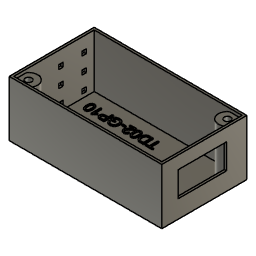
TD02-GP10 (Autodesk Fusion 360 archive; units mm, degrees)
design "boite"
Autodesk Fusion 360 part; units mm, degrees
note: some values were not read from the file. Chosen so that the rebuilt part matches the saved one: that a step has no effect; which face or edge a step refers to; which pieces of a blend or face edit are solid. Set by a fixed rule: which sketch regions a step uses.
sketch "Sketch1" plane through (0, 0, 0) normal (0, 0, 1) x (1, 0, 0)
  line L0 (-39.5, 22) -> (39.5, 22)
  line L1 (39.5, 22) -> (39.5, -22)
  line L2 (39.5, -22) -> (-39.5, -22)
  line L3 (-39.5, -22) -> (-39.5, 22)
  line L4 (-39.5, 22) -> (39.5, -22) construction
  line L5 (39.5, 22) -> (-39.5, -22) construction
  line L6 (38.3, -20.8) -> (-38.3, -20.8)
  line L7 (-38.3, -20.8) -> (-38.3, 20.8)
  line L8 (-38.3, 20.8) -> (38.3, 20.8)
  line L9 (38.3, 20.8) -> (38.3, -20.8)
  line L10 (-37.5, 20) -> (37.5, 20) construction
  line L11 (37.5, 20) -> (37.5, -20) construction
  line L12 (37.5, -20) -> (-37.5, -20) construction
  line L13 (-37.5, -20) -> (-37.5, 20) construction
  line L14 (-37.5, 20) -> (37.5, -20) construction
  line L15 (37.5, 20) -> (-37.5, -20) construction
  line L16 (-37.5, 20) -> (-34.5, 20) construction
  line L17 (-34.5, 20) -> (-34.5, 17) construction
  line L18 (-34.5, 17) -> (-37.5, 17) construction
  line L19 (-37.5, 17) -> (-37.5, 20) construction
  circle A0 centre (-34.5, 17) radius 2.9
  line L20 (37.5, -20) -> (34.5, -20) construction
  line L21 (34.5, -20) -> (34.5, -17) construction
  line L22 (34.5, -17) -> (37.5, -17) construction
  line L23 (37.5, -17) -> (37.5, -20) construction
  circle A1 centre (34.5, -17) radius 2.9
  circle A2 centre (-34.5, 17) radius 3.7
  circle A3 centre (34.5, -17) radius 3.7
  circle A4 centre (-34.5, 17) radius 1.7
  circle A5 centre (34.5, -17) radius 1.7
  line L24 (20, 0) -> (2.5, 0)
  circle A6 centre (-34.5, -17) radius 3.7
  circle A7 centre (-34.5, -17) radius 2.9
  circle A8 centre (-34.5, -17) radius 1.7
  circle A9 centre (34.5, 17) radius 3.7
  circle A10 centre (34.5, 17) radius 2.9
  circle A11 centre (34.5, 17) radius 1.7
  circle A12 centre (34.5, 17) radius 4.7
  circle A13 centre (-34.5, -17) radius 4.7
  dimension "d1" = 79
  dimension "d2" = 44
  dimension "d3" = 1.2
  dimension "d4" = 75
  dimension "d5" = 40
  dimension "d6" = 3
  dimension "d7" = 3
  dimension "d8" = 5.8
  dimension "d10" = 3
  dimension "d11" = 3
  dimension "d12" = 5.8
  dimension "d32" = 0.8
  dimension "d33" = 0.8
  dimension "d44" = 3.4
  dimension "d45" = 3.4
  dimension "d90" = 1
  dimension "d91" = 1
  constraint horizontal L0
  constraint perpendicular L0 L1
  constraint parallel L0 L2
  constraint parallel L1 L3
  constraint coincident L4 origin
  constraint coincident L5 origin
  constraint horizontal L10
  constraint perpendicular L10 L11
  constraint parallel L10 L12
  constraint parallel L11 L13
  constraint coincident L14 origin
  constraint coincident L15 origin
  constraint horizontal L16
  constraint vertical L17
  constraint horizontal L18
  constraint vertical L19
  constraint coincident L17.end L18.start
  constraint horizontal L20
  constraint vertical L21
  constraint horizontal L22
  constraint vertical L23
  constraint coincident L21.end L22.start
  constraint concentric A0 A4
  constraint concentric A1 A5
  constraint symmetric A0 L24 A7
  constraint symmetric A1 L24 A10
  constraint symmetric A2 L24 A6
  constraint symmetric A3 L24 A9
  constraint symmetric A4 L24 A8
  constraint symmetric A5 L24 A11
  measures "d1" distance of L0.start L0.end
  measures "d2" distance of L0.start L2.end
  measures "d4" distance of L11.end L12.end
  measures "d5" distance of L10.start L12.end
  measures "d6" distance of L10.start L16.end
  measures "d7" distance of L16.end L17.end
  measures "d8" diameter of A0
  measures "d10" distance of L11.end L22.end
  measures "d11" distance of L21.end L22.end
  measures "d12" diameter of A1
  measures "d44" diameter of A4
  measures "d45" diameter of A5
extrude "Extrude7" [no effect]
extrude "Extrude9" add sketch "Sketch1" against normal blind 1.2 contours L0 L1 L2 L3 | L6 L7 L8 L9 A12 A13 | L6 A13 | L6 L7 A13 | L8 L9 A12 | L9 A12 | L6 L7 A13 | L8 L9 A12 | L8 A12 | L7 A13 | A2 | A3 | A6 | A7 | A8 | A9 | A10 | A11
extrude "Extrude10" add sketch "Sketch1" along normal blind 27.6 contours L0 L1 L2 L3 | L6 A13 | L9 A12 | L8 A12 | L7 A13 | A0 | A1 | A2 | A3 | A4 | A5
extrude "Extrude11" cut sketch "Sketch1" along normal blind 21.6 contours A1 | A5
extrude "Extrude12" cut sketch "Sketch1" along normal blind 22.2 contours A0 | A4
extrude "Extrude13" cut 1 faces at (33.7592, -18.0865, 21.6) along direction (0, 0, 1) blind 0.6
extrude "Extrude14" cut sketch "Sketch1" along normal blind 40 contours A5
extrude "Extrude15" cut sketch "Sketch1" along normal blind 34 contours A4
extrude "Extrude16" cut sketch "Sketch1" along normal mid plane 100 contours A11
extrude "Extrude17" add sketch "Sketch1" along normal blind 27.6 contours A9 | A10
extrude "Extrude18" cut sketch "Sketch1" against normal blind 6 contours A10
extrude "Extrude19" cut sketch "Sketch1" along normal blind 22.2 contours A10
extrude "Extrude20" cut sketch "Sketch1" along normal mid plane 92 contours A8
extrude "Extrude21" add sketch "Sketch1" along normal blind 26.6 contours A6 | A7
extrude "Extrude22" cut sketch "Sketch1" along normal blind 22.2 contours A7
extrude "Extrude23" cut sketch "Sketch1" against normal blind 3 contours A7
delete_face "DeleteFace1" 1 faces at (-32.0171, 16.7715, 22.2)
delete_face "DeleteFace2" 6 faces at (-30.8184, 17.3684, 10.2757) (-30.8184, 17.3684, 19.4757) (-31.0912, 16.6721, 27.6) (-31.6144, 17.2887, 25.8) (-31.6144, 17.2887, 17.6757) (-31.6144, 17.2887, 10.2757)
delete_face "DeleteFace3" 1 faces at (-31.6036, 16.8554, -0.8)
delete_face "DeleteFace4" 1 faces at (38.1954, -17.1844, 18.4)
delete_face "DeleteFace5" 1 faces at (37.3964, -17.1446, -0.8)
sketch "Sketch3" plane through (39.5, 0, 0) normal (1, 0, 0) x (0, 1, 0)
  line L0 (-22, 27.6) -> (-22, -1.2) construction
  line L1 (-22, -1.2) -> (22, -1.2) construction
  line L2 (22, -1.2) -> (22, 27.6) construction
  line L3 (22, 27.6) -> (-22, 27.6) construction
  line L4 (-22, 27.6) -> (-9, 27.6) construction
  line L5 (-9, 27.6) -> (-9, 16.6) construction
  line L6 (-9, 16.6) -> (-22, 16.6) construction
  line L7 (-22, 16.6) -> (-22, 27.6) construction
  circle A0 centre (-12, 19.8) radius 4.3863
  line L8 (-7.9908, 18.0207) -> (-11.9971, 8.9935)
  line L9 (-11.9971, 8.9935) -> (-16.0083, 18.0185)
  dimension "d66" = 13
  dimension "d67" = 11
  dimension "d68" = 9.8762
  constraint horizontal L4
  constraint vertical L5
  constraint horizontal L6
  constraint vertical L7
  constraint coincident L0.start L3.end
  constraint coincident L5.end A0
  constraint coincident A0 L8.start
  constraint coincident A0 L9.end
  constraint tangent A0 L9
  constraint tangent A0 L8
  measures "d66" distance of L0.start L4.end
  measures "d67" distance of L4.end L5.end
  measures "d68" distance of L8.start L8.end
move_body "Move1" bodies 1 to x (1, 0, 0) y (0, 1, 0) z (0, 0, 1) at (0, -5.5, 0)
move_body "Move2" bodies 1 to x (1, 0, 0) y (0, 1, 0) z (0, 0, 1) at (0, 3, 0)
extrude "Extrude24" cut sketch "Sketch3" against normal blind 14
extrude "Extrude25" cut 1 faces at (-31.4868, -19.7683, 26.6) along direction (0, 0, -1) blind 0.6
extrude "Extrude26" cut 1 faces at (37.5132, 14.2317, 27.6) along direction (0, 0, -1) blind 1.6
delete_face "DeleteFace6" 2 faces at (39.1, -16.1636, 18.4201) (39.1, -9.3262, 15.0116)
sketch "Sketch4" plane through (39.5, 0, 0) normal (1, 0, 0) x (0, 1, 0)
  line L0 (19.5, 27.6) -> (-24.5, 27.6)
  line L1 (-24.5, 27.6) -> (-24.5, -1.2)
  line L2 (-24.5, -1.2) -> (19.5, -1.2)
  line L3 (19.5, -1.2) -> (19.5, 27.6)
  line L4 (9, 8) -> (-16, 8)
  line L5 (-16, 8) -> (-16, 21)
  line L6 (-16, 21) -> (9, 21)
  line L7 (9, 21) -> (9, 8)
  constraint horizontal L4
  constraint vertical L5
  constraint horizontal L6
  constraint vertical L7
extrude "Extrude27" cut sketch "Sketch4" against normal blind 16 contours L4 L5 L6 L7
sketch "Sketch5" plane through (0, 0, -1.2) normal (0, 0, -1) x (1, 0, 0)
  circle A0 centre (-34.5, 19.5) radius 2.9
  circle A1 centre (34.5, -14.5) radius 2.9
  line L0 (39.5, 24.5) -> (-39.5, 24.5)
  line L1 (-39.5, 24.5) -> (-39.5, -19.5)
  line L2 (-39.5, -19.5) -> (39.5, -19.5)
  line L3 (39.5, -19.5) -> (39.5, 24.5)
  circle A2 centre (23, 13) radius 7.6158
extrude "Extrude28" cut sketch "Sketch5" against normal blind 5 contours A2
sketch "Sketch6" plane through (0, 0, 0) normal (0, 0, 1) x (-1, 0, 0)
  circle A0 centre (-23, 13) radius 7.6158
  circle A1 centre (34.5, 19.5) radius 3.7
  circle A2 centre (-34.5, -14.5) radius 3.7
  line L0 (38.3, -18.3) -> (38.3, 23.3)
  line L1 (38.3, 23.3) -> (-38.3, 23.3)
  line L2 (-38.3, 23.3) -> (-38.3, -18.3)
  line L3 (-38.3, -18.3) -> (38.3, -18.3)
  line L4 (-3.0028, -22.2598) -> (29.9972, -22.2598) construction
  line L5 (29.9972, -22.2598) -> (29.9972, -7.2598) construction
  line L6 (29.9972, -7.2598) -> (-3.0028, -7.2598) construction
  line L7 (-3.0028, -7.2598) -> (-3.0028, -22.2598) construction
  dimension "d79" = 5
  text T0 "TD02-GP10\n" font "Arial" height 5 align left top in box 33 x 15 at (-3.0028, -22.2598) x (1, 0) y (0, 1) spacing 1
extrude "Extrude29" add sketch "Sketch6" along normal blind 0.4 text T0
sketch "Sketch7" plane through (-39.5, 0, 0) normal (-1, 0, 0) x (0, -1, 0)
  line L0 (-19.5, 27.6) -> (-19.5, -1.2)
  line L1 (-19.5, -1.2) -> (24.5, -1.2)
  line L2 (24.5, -1.2) -> (24.5, 27.6)
  line L3 (24.5, 27.6) -> (-19.5, 27.6)
  line L4 (12, 2) -> (9.8, 2)
  line L5 (9.8, 2) -> (9.8, 4.2)
  line L6 (9.8, 4.2) -> (12, 4.2)
  line L7 (12, 4.2) -> (12, 2)
  line L8 (0, 2) -> (-2.2, 2)
  line L9 (0, 4.2) -> (0, 2)
  line L10 (-2.2, 4.2) -> (0, 4.2)
  line L11 (-2.2, 2) -> (-2.2, 4.2)
  line L12 (-12, 2) -> (-14.2, 2)
  line L13 (-12, 4.2) -> (-12, 2)
  line L14 (-14.2, 4.2) -> (-12, 4.2)
  line L15 (-14.2, 2) -> (-14.2, 4.2)
  line L16 (12, 10.5) -> (9.8, 10.5)
  line L17 (12, 12.7) -> (12, 10.5)
  line L18 (9.8, 12.7) -> (12, 12.7)
  line L19 (9.8, 10.5) -> (9.8, 12.7)
  line L20 (0, 10.5) -> (-2.2, 10.5)
  line L21 (0, 12.7) -> (0, 10.5)
  line L22 (-2.2, 12.7) -> (0, 12.7)
  line L23 (-2.2, 10.5) -> (-2.2, 12.7)
  line L24 (-12, 10.5) -> (-14.2, 10.5)
  line L25 (-12, 12.7) -> (-12, 10.5)
  line L26 (-14.2, 12.7) -> (-12, 12.7)
  line L27 (-14.2, 10.5) -> (-14.2, 12.7)
  line L28 (12, 19) -> (9.8, 19)
  line L29 (12, 21.2) -> (12, 19)
  line L30 (9.8, 21.2) -> (12, 21.2)
  line L31 (9.8, 19) -> (9.8, 21.2)
  line L32 (0, 19) -> (-2.2, 19)
  line L33 (0, 21.2) -> (0, 19)
  line L34 (-2.2, 21.2) -> (0, 21.2)
  line L35 (-2.2, 19) -> (-2.2, 21.2)
  line L36 (-12, 19) -> (-14.2, 19)
  line L37 (-12, 21.2) -> (-12, 19)
  line L38 (-14.2, 21.2) -> (-12, 21.2)
  line L39 (-14.2, 19) -> (-14.2, 21.2)
  dimension "d82" = 2.2
  dimension "d83" = 2.2
  dimension "d86" = -24
  dimension "d87" = 17
  constraint horizontal L4
  constraint vertical L5
  constraint horizontal L6
  constraint vertical L7
  measures "d82" distance of L4.start L6.end
  measures "d83" distance of L4.start L4.end
extrude "Extrude30" cut sketch "Sketch7" against normal blind 26 contours L4 L5 L6 L7 | L8 L9 L10 L11 | L12 L13 L14 L15 | L16 L17 L18 L19 | L20 L21 L22 L23 | L24 L25 L26 L27 | L28 L29 L30 L31 | L32 L33 L34 L35 | L36 L37 L38 L39
move_body "Move3" bodies 1 to x (1, 0, 0) y (0, 1, 0) z (0, 0, 1) at (0, 2.5, 0)
extrude "Extrude31" add sketch "Sketch1" along normal blind 26 contours L6 L7 A13 picked at (-37.7879, -14.1407)
extrude "Extrude32" add sketch "Sketch1" along normal blind 26 contours L8 L9 A12 picked at (30.1903, 17.6511)
sketch "Sketch8" plane through (0, 0, 22.2) normal (0, 0, -1) x (1, 0, 0)
  circle A0 centre (34.5, -17) radius 1.7
  circle A1 centre (34.5, -17) radius 2.9
  line L0 (31.6, -14.1) -> (37.4, -14.1)
  line L1 (37.4, -14.1) -> (37.4, -19.9)
  line L2 (37.4, -19.9) -> (31.6, -19.9)
  line L3 (31.6, -19.9) -> (31.6, -14.1)
  line L4 (31.6, -14.1) -> (37.4, -19.9) construction
  line L5 (37.4, -14.1) -> (31.6, -19.9) construction
  line L6 (32.8, -15.3) -> (36.2, -15.3)
  line L7 (36.2, -15.3) -> (36.2, -18.7)
  line L8 (36.2, -18.7) -> (32.8, -18.7)
  line L9 (32.8, -18.7) -> (32.8, -15.3)
  line L10 (32.8, -15.3) -> (36.2, -18.7) construction
  line L11 (36.2, -15.3) -> (32.8, -18.7) construction
  line L12 (36.2, -18.7) -> (37.4, -18.7)
  line L13 (32.8, -18.7) -> (31.6, -18.7)
  line L14 (32.8, -15.3) -> (31.6, -15.3)
  line L15 (36.2, -15.3) -> (37.4, -15.3)
  line L16 (36.2, -15.3) -> (36.2, -14.1)
  line L17 (32.8, -15.3) -> (32.8, -14.1)
  line L18 (32.8, -18.7) -> (32.8, -19.9)
  line L19 (36.2, -18.7) -> (36.2, -19.9)
  point P0 (34.5, -17)
  point P1 (34.5, -17)
  constraint horizontal L0
  constraint perpendicular L0 L1
  constraint parallel L0 L2
  constraint parallel L1 L3
  constraint coincident L4 P1
  constraint coincident L5 P1
  constraint coincident P0 A0.centre
  constraint horizontal L6
  constraint perpendicular L6 L7
  constraint parallel L6 L8
  constraint parallel L7 L9
  constraint coincident L10 P1
  constraint coincident L11 P1
  constraint coincident L4 L6.start
  constraint coincident P1 P0
  constraint coincident L1 L12.end
  constraint perpendicular L1 L12
  constraint coincident L3 L13.end
  constraint perpendicular L3 L13
  constraint coincident L3 L14.end
  constraint perpendicular L3 L14
  constraint coincident L1 L15.end
  constraint perpendicular L1 L15
  constraint coincident L0 L16.end
  constraint perpendicular L0 L16
  constraint coincident L0 L17.end
  constraint perpendicular L0 L17
  constraint coincident L2 L18.end
  constraint perpendicular L2 L18
  constraint coincident L2 L19.end
  constraint perpendicular L2 L19
  constraint tangent A0 L6
  constraint tangent A0 L9
extrude "Extrude33" add sketch "Sketch8" along normal blind 0.4 contours A1 L9 L13 L14
extrude "Extrude34" add sketch "Sketch8" along normal blind 0.4 contours A1 L14 L17 | A1 L13 L18
extrude "Extrude35" add sketch "Sketch8" along normal blind 0.4 contours A1 L7 L12 L15 | A1 L15 L16 | A1 L12 L19 | A1 L9 L13 L14 | A1 L14 L17 | A1 L13 L18
extrude "Extrude36" add sketch "Sketch8" along normal blind 0.3 contours A1 L7 L12 L15 | A1 L6 L16 L17 | A1 L8 L18 L19 | A1 L15 L16 | A1 L12 L19 | A1 L9 L13 L14 | A1 L14 L17 | A1 L13 L18
sketch "Sketch9" plane through (0, 0, 22.2) normal (0, 0, -1) x (1, 0, 0)
  circle A0 centre (-34.5, 17) radius 1.7
  circle A1 centre (-34.5, 17) radius 2.9
  line L0 (-36.2, 18.7) -> (-32.8, 18.7)
  line L1 (-32.8, 18.7) -> (-32.8, 15.3)
  line L2 (-32.8, 15.3) -> (-36.2, 15.3)
  line L3 (-36.2, 15.3) -> (-36.2, 18.7)
  line L4 (-36.2, 18.7) -> (-32.8, 15.3) construction
  line L5 (-32.8, 18.7) -> (-36.2, 15.3) construction
  line L6 (-37.4, 19.9) -> (-31.6, 19.9)
  line L7 (-31.6, 19.9) -> (-31.6, 14.1)
  line L8 (-31.6, 14.1) -> (-37.4, 14.1)
  line L9 (-37.4, 14.1) -> (-37.4, 19.9)
  line L10 (-37.4, 19.9) -> (-31.6, 14.1) construction
  line L11 (-31.6, 19.9) -> (-37.4, 14.1) construction
  line L12 (-36.2, 18.7) -> (-37.4, 18.7)
  line L13 (-36.2, 19.9) -> (-36.2, 18.7)
  line L14 (-32.8, 18.7) -> (-31.6, 18.7)
  line L15 (-32.8, 19.9) -> (-32.8, 14.1)
  line L16 (-37.4, 15.3) -> (-31.6, 15.3)
  line L17 (-36.2, 15.3) -> (-36.2, 14.1)
  point P0 (-34.5, 17)
  point P1 (-34.5, 17)
  constraint horizontal L0
  constraint perpendicular L0 L1
  constraint parallel L0 L2
  constraint parallel L1 L3
  constraint coincident L4 P1
  constraint coincident L5 P1
  constraint coincident P0 A0.centre
  constraint horizontal L6
  constraint perpendicular L6 L7
  constraint parallel L6 L8
  constraint parallel L7 L9
  constraint coincident L10 P1
  constraint coincident L11 P1
  constraint coincident P1 P0
  constraint tangent A0 L0
  constraint tangent A0 L3
  constraint tangent A1 L6
  constraint tangent A1 L9
  constraint coincident L9 L12.end
  constraint perpendicular L9 L12
  constraint coincident L6 L13.start
  constraint perpendicular L0 L13
  constraint coincident L7 L14.end
  constraint perpendicular L7 L14
  constraint coincident L6 L15.start
  constraint coincident L8 L15.end
  constraint perpendicular L8 L15
  constraint coincident L9 L16.start
  constraint coincident L7 L16.end
  constraint perpendicular L7 L16
  constraint coincident L8 L17.end
  constraint perpendicular L8 L17
extrude "Extrude37" add sketch "Sketch9" along normal blind 0.4 contours A1 L1 L14 L15 L16 | A1 L14 L15 | A1 L15 L16 | A1 L3 L12 L16 | A1 L12 L13 | A1 L16 L17
extrude "Extrude38" add sketch "Sketch9" along normal blind 0.3 contours A1 L0 L13 L15 | A1 L2 L15 L16 L17
delete_face "DeleteFace7" 1 faces at (30.5172, -9.2783, -0.8)
hole "Hole1" at (30.1371, -11.9835, -1.2) direction (0, 0, 1) diameter 12 depth 2 tip angle 118

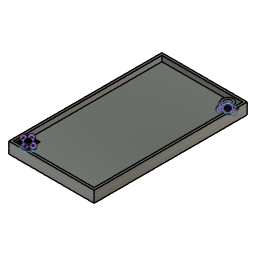
design "base"
Autodesk Fusion 360 part; units mm, degrees
sketch "Sketch1" plane through (0, 0, 0) normal (0, 0, 1) x (1, 0, 0)
  line L0 (22, -39.5) -> (-22, -39.5)
  line L1 (-22, -39.5) -> (-22, 39.5)
  line L2 (-22, 39.5) -> (22, 39.5)
  line L3 (22, 39.5) -> (22, -39.5)
  line L4 (22, -39.5) -> (-22, 39.5) construction
  line L5 (-22, -39.5) -> (22, 39.5) construction
  line L6 (-20.8, -38.3) -> (-20.8, 38.3)
  line L7 (-20.8, 38.3) -> (20.8, 38.3)
  line L8 (20.8, 38.3) -> (20.8, -38.3)
  line L9 (20.8, -38.3) -> (-20.8, -38.3)
  line L10 (20, 37.5) -> (-20, 37.5) construction
  line L11 (-20, 37.5) -> (-20, -37.5) construction
  line L12 (-20, -37.5) -> (20, -37.5) construction
  line L13 (20, -37.5) -> (20, 37.5) construction
  line L14 (20, 37.5) -> (-20, -37.5) construction
  line L15 (-20, 37.5) -> (20, -37.5) construction
  line L16 (20, 37.5) -> (17, 37.5) construction
  line L17 (17, 37.5) -> (17, 34.5) construction
  line L18 (17, 34.5) -> (20, 34.5) construction
  line L19 (20, 34.5) -> (20, 37.5) construction
  circle A0 centre (17, 34.5) radius 1.7
  line L20 (-20, -37.5) -> (-17, -37.5) construction
  line L21 (-17, -37.5) -> (-17, -34.5) construction
  line L22 (-17, -34.5) -> (-20, -34.5) construction
  line L23 (-20, -34.5) -> (-20, -37.5) construction
  circle A1 centre (-17, -34.5) radius 1.7
  circle A2 centre (17, 34.5) radius 2.9
  circle A3 centre (-17, -34.5) radius 2.9
  line L24 (0, -38.3) -> (0, 38.3)
  circle A4 centre (17, -34.5) radius 1.7
  circle A5 centre (17, -34.5) radius 2.9
  circle A6 centre (-17, 34.5) radius 2.9
  circle A7 centre (-17, 34.5) radius 1.7
  dimension "d6" = 79
  dimension "d7" = 44
  dimension "d8" = 1.2
  dimension "d9" = 40
  dimension "d10" = 75
  dimension "d11" = 3
  dimension "d12" = 3
  dimension "d13" = 3.4
  dimension "d14" = 3
  dimension "d15" = 3
  dimension "d16" = 3.4
  dimension "d17" = 1.2
  dimension "d18" = 1.2
  constraint horizontal L0
  constraint perpendicular L0 L1
  constraint parallel L0 L2
  constraint parallel L1 L3
  constraint coincident L4 origin
  constraint coincident L5 origin
  constraint horizontal L10
  constraint perpendicular L10 L11
  constraint parallel L10 L12
  constraint parallel L11 L13
  constraint coincident L14 origin
  constraint coincident L15 origin
  constraint horizontal L16
  constraint vertical L17
  constraint horizontal L18
  constraint vertical L19
  constraint coincident L17.end L18.start
  constraint horizontal L20
  constraint vertical L21
  constraint horizontal L22
  constraint vertical L23
  constraint coincident L21.end L22.start
  constraint midpoint L9 L24.start
  constraint midpoint L7 L24.end
  constraint symmetric A0 L24 A7
  constraint symmetric A1 L24 A4
  constraint symmetric A2 L24 A6
  constraint symmetric A3 L24 A5
  measures "d6" distance of L0.end L1.end
  measures "d7" distance of L1.end L2.end
  measures "d9" distance of L11.end L12.end
  measures "d10" distance of L10.start L12.end
  measures "d11" distance of L10.start L18.end
  measures "d12" distance of L17.end L18.end
  measures "d13" diameter of A0
  measures "d14" distance of L11.end L20.end
  measures "d15" distance of L20.end L21.end
  measures "d16" diameter of A1
extrude "Extrude1" add sketch "Sketch1" against normal blind 3.4 contours L0 L1 L2 L3 | L6 L7 L9 L24 | L7 L8 L9 L24 | A4 | A5 | A6 | A7
extrude "Extrude2" add sketch "Sketch1" against normal blind 3.4 contours A3
extrude "Extrude3" add sketch "Sketch1" against normal blind 3.4 contours A2
extrude "Extrude4" add sketch "Sketch1" along normal blind 1.2 contours A2
extrude "Extrude5" add sketch "Sketch1" along normal blind 1.2 contours A3
extrude "Extrude6" add sketch "Sketch1" along normal blind 2.8 contours L0 L1 L2 L3
extrude "Extrude7" cut 1 faces at (7.5605, -13.2761, -3.4) along direction (0, 0, 1) blind 0.4
ref_plane "WorkPlane1" through (0, 0, 2.8) normal (0, 0, 1) x (1, 0, 0)
extrude "Extrude8" add 2 faces at (-14.5171, -34.7285, 1.2) (19.4829, 34.2715, 1.2) along direction (0, 0, 1) blind 1.6
sketch "Sketch3" plane through (0, 0, -3) normal (0, 0, -1) x (1, 0, 0)
  circle A0 centre (17, -34.5) radius 1.7
  circle A1 centre (-17, 34.5) radius 1.7
  line L0 (-22, -39.5) -> (22, -39.5)
  line L1 (22, -39.5) -> (22, 39.5)
  line L2 (22, 39.5) -> (-22, 39.5)
  line L3 (-22, 39.5) -> (-22, -39.5)
  line L4 (19.9499, -34.473) -> (18.4516, -31.9318)
  line L5 (18.4516, -31.9318) -> (15.5017, -31.9588)
  line L6 (15.5017, -31.9588) -> (14.0501, -34.527)
  line L7 (14.0501, -34.527) -> (15.5484, -37.0682)
  line L8 (15.5484, -37.0682) -> (18.4983, -37.0412)
  line L9 (18.4983, -37.0412) -> (19.9499, -34.473)
  line L10 (-15.1571, 32.1964) -> (-14.0836, 34.9442)
  line L11 (-14.0836, 34.9442) -> (-15.9265, 37.2477)
  line L12 (-15.9265, 37.2477) -> (-18.8429, 36.8036)
  line L13 (-18.8429, 36.8036) -> (-19.9164, 34.0558)
  line L14 (-19.9164, 34.0558) -> (-18.0735, 31.7523)
  line L15 (-18.0735, 31.7523) -> (-15.1571, 32.1964)
  point P0 (17, -34.5)
  point P1 (-17, 34.5)
  dimension "d36" = 2.95
  dimension "d37" = 2.95
  constraint coincident P0 A0.centre
  constraint coincident P1 A1.centre
  measures "d36" distance of L4.start P0
  measures "d37" distance of L10.start P1
extrude "Extrude9" cut sketch "Sketch3" against normal blind 2.5 contours L10 L11 L12 L13 L14 L15
extrude "Extrude10" cut sketch "Sketch3" against normal blind 2.5 contours L4 L5 L6 L7 L8 L9
sketch "Sketch4" plane through (0, 0, -0.5) normal (0, 0, -1) x (1, 0, 0)
  circle A0 centre (17, -34.5) radius 1.7
  line L0 (18.4983, -37.0412) -> (19.9499, -34.473)
  line L1 (19.9499, -34.473) -> (18.4516, -31.9318)
  line L2 (18.4516, -31.9318) -> (15.5017, -31.9588)
  line L3 (15.5017, -31.9588) -> (14.0501, -34.527)
  line L4 (14.0501, -34.527) -> (15.5484, -37.0682)
  line L5 (15.5484, -37.0682) -> (18.4983, -37.0412)
  line L6 (-19.9164, 31.7523) -> (-14.0836, 31.7523)
  line L7 (-14.0836, 31.7523) -> (-14.0836, 37.2477)
  line L8 (-14.0836, 37.2477) -> (-19.9164, 37.2477)
  line L9 (-19.9164, 37.2477) -> (-19.9164, 31.7523)
  line L10 (-19.9164, 31.7523) -> (-14.0836, 37.2477) construction
  line L11 (-14.0836, 31.7523) -> (-19.9164, 37.2477) construction
  line L12 (-15.3, 32.8) -> (-18.7, 32.8)
  line L13 (-18.7, 32.8) -> (-18.7, 36.2)
  line L14 (-18.7, 36.2) -> (-15.3, 36.2)
  line L15 (-15.3, 36.2) -> (-15.3, 32.8)
  line L16 (-15.3, 32.8) -> (-18.7, 36.2) construction
  line L17 (-18.7, 32.8) -> (-15.3, 36.2) construction
  circle A1 centre (-17, 34.5) radius 1.7
  line L18 (-15.3, 32.8) -> (-15.3, 31.7523)
  line L19 (-15.3, 32.8) -> (-14.0836, 32.8)
  line L20 (-15.3, 36.2) -> (-15.3, 37.2477)
  line L21 (-15.3, 36.2) -> (-14.0836, 36.2)
  line L22 (-18.7, 36.2) -> (-18.7, 37.2477)
  line L23 (-18.7, 36.2) -> (-19.9164, 36.2)
  line L24 (-18.7, 32.8) -> (-18.7, 31.7523)
  line L25 (-18.7, 32.8) -> (-19.9164, 32.8)
  point P0 (-17, 34.5)
  point P1 (-15.9265, 37.2477)
  point P2 (-19.9164, 34.0558)
  point P3 (-18.0735, 31.7523)
  point P4 (-14.0836, 34.9442)
  point P5 (-17, 34.5)
  constraint horizontal L6
  constraint perpendicular L6 L7
  constraint parallel L6 L8
  constraint parallel L7 L9
  constraint coincident L10 P5
  constraint coincident L11 P5
  constraint coincident L8 P1
  constraint coincident L9 P2
  constraint coincident L6 P3
  constraint coincident L7 P4
  constraint horizontal L12
  constraint perpendicular L12 L13
  constraint parallel L12 L14
  constraint parallel L13 L15
  constraint coincident L16 P5
  constraint coincident L17 P5
  constraint coincident P5 P0
  constraint tangent L12 A1
  constraint tangent L13 A1
  constraint coincident L6 L18.end
  constraint perpendicular L6 L18
  constraint coincident L7 L19.end
  constraint perpendicular L7 L19
  constraint coincident L8 L20.end
  constraint perpendicular L8 L20
  constraint coincident L7 L21.end
  constraint perpendicular L7 L21
  constraint coincident L8 L22.end
  constraint perpendicular L8 L22
  constraint coincident L9 L23.end
  constraint perpendicular L9 L23
  constraint coincident L6 L24.end
  constraint perpendicular L6 L24
  constraint coincident L9 L25.end
  constraint perpendicular L9 L25
extrude "Extrude11" add sketch "Sketch4" along normal blind 0.4 contours L6 L9 L24 L25 | L9 L13 L23 L25 | L6 L7 L18 L19 | L8 L9 L22 L23 | L7 L15 L19 L21 | L7 L8 L20 L21
extrude "Extrude12" add sketch "Sketch4" along normal blind 0.3 contours L6 L12 L18 L24 | L8 L14 L20 L22
sketch "Sketch5" plane through (0, 0, -3) normal (0, 0, -1) x (1, 0, 0)
  line L0 (15.3, -32.8) -> (18.7, -32.8)
  line L1 (18.7, -32.8) -> (18.7, -36.227)
  line L2 (18.7, -36.227) -> (15.3, -36.227)
  line L3 (15.3, -36.227) -> (15.3, -32.8)
  line L4 (15.3, -32.8) -> (18.7, -36.227) construction
  line L5 (18.7, -32.8) -> (15.3, -36.227) construction
  line L6 (14.0501, -31.9588) -> (19.9499, -31.9588)
  line L7 (19.9499, -31.9588) -> (19.9499, -37.0682)
  line L8 (19.9499, -37.0682) -> (14.0501, -37.0682)
  line L9 (14.0501, -37.0682) -> (14.0501, -31.9588)
  line L10 (14.0501, -31.9588) -> (19.9499, -37.0682) construction
  line L11 (19.9499, -31.9588) -> (14.0501, -37.0682) construction
  circle A0 centre (17, -34.5) radius 1.7
  line L12 (15.3, -32.8) -> (15.3, -31.9588)
  line L13 (15.3, -31.9588) -> (15.3, -32.8)
  line L14 (18.7, -32.8) -> (18.7, -31.9588)
  line L15 (18.7, -31.9588) -> (18.7, -32.8)
  line L16 (19.9499, -32.8) -> (18.7, -32.8)
  line L17 (18.7, -35.9857) -> (18.7, -37.0682)
  line L18 (18.7, -36.227) -> (19.9499, -36.227)
  line L19 (15.3, -36.227) -> (15.3, -37.0682)
  line L20 (15.3, -36.227) -> (14.0501, -36.227)
  line L21 (15.3, -32.8) -> (14.0501, -32.8)
  point P0 (17, -34.5135)
  point P1 (17, -34.5135)
  point P2 (15.5017, -31.9588)
  point P3 (14.0501, -34.527)
  point P4 (15.5484, -37.0682)
  point P5 (19.9499, -34.473)
  constraint horizontal L0
  constraint perpendicular L0 L1
  constraint parallel L0 L2
  constraint parallel L1 L3
  constraint coincident L4 P1
  constraint coincident L5 P1
  constraint horizontal L6
  constraint perpendicular L6 L7
  constraint parallel L6 L8
  constraint parallel L7 L9
  constraint coincident L10 P1
  constraint coincident L11 P1
  constraint coincident P1 P0
  constraint coincident L6 P2
  constraint coincident L9 P3
  constraint coincident L8 P4
  constraint coincident L7 P5
  constraint tangent L0 A0
  constraint tangent L3 A0
  constraint coincident L6 L12.end
  constraint perpendicular L6 L12
  constraint coincident L6 L14.end
  constraint perpendicular L6 L14
  constraint coincident L7 L16.start
  constraint perpendicular L15 L16
  constraint coincident L1 L17.start
  constraint coincident L10 L17.start
  constraint coincident L8 L17.end
  constraint perpendicular L8 L17
  constraint coincident L7 L18.end
  constraint perpendicular L7 L18
  constraint coincident L8 L19.end
  constraint perpendicular L8 L19
  constraint coincident L9 L20.end
  constraint perpendicular L9 L20
  constraint coincident L9 L21.end
  constraint perpendicular L9 L21
move_body "Move1" bodies 1 to x (1, 0, 0) y (0, 1, 0) z (0, 0, 1) at (0, 0, -3)
extrude "Extrude13" add sketch "Sketch5" along normal blind 0.9 contours L0 L6 L12 L13 L14 L15 | L6 L9 L12 L13 L21 | L6 L7 L14 L15 L16 | L2 L8 L17 L19 | L8 L9 L19 L20 | L7 L8 L17 L18
extrude "Extrude14" add sketch "Sketch5" along normal blind 0.8 contours L3 L9 L20 L21 | L1 L7 L16 L17 L18
